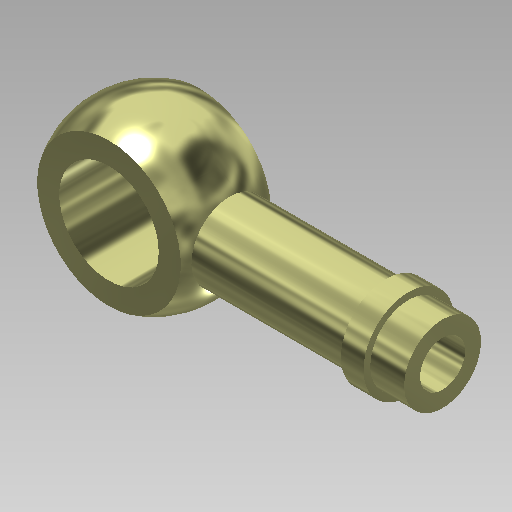
# Autodesk Inventor part: fuel_inlet
Saved by Autodesk Inventor 2018.1 (Build 221171000, 171)
## iProperties
Created: 2013-08-26
Part Number: fuel_inlet
Material: Generic
Document SubType Name: Modeling
Designer: Konstantin
Density: 1 g/cm^3
Appearance: Default
Mass: 0.152735 g
Surface Area: 3.51801 cm^2
Volume: 0.152735 cm^3
Author: Konstantin
Autodesk Inventor part; units mm, degrees
ref_plane "YZ Plane" through (0, 0, 0) normal (1, 0, 0) x (0, 1, 0)
ref_plane "XZ Plane" through (0, 0, 0) normal (0, 1, 0) x (-1, 0, 0)
ref_plane "XY Plane" through (0, 0, 0) normal (0, 0, 1) x (1, 0, 0)
sketch "Sketch2" plane through (0, 0, 0) normal (0, 0, 1) x (1, 0, 0)
  arc A0 (0, -3.75) -> (0, 3.75) centre (0, 0) ccw
  line L0 (0, -3.75) -> (0, 3.75)
  constraints: 2 end point, 2 point on circle, 1 centre point, 1 midpoint, 1 vertical, 1 other
revolve "Revolution2" add sketch "Sketch2" angle 360 about axis through (0, -3.75, 0) along (0, 1, 0)
sketch "Sketch3" plane through (0, 0, 0) normal (1, 0, 0) x (0, 1, 0)
  line L0 (4.6089, 2) -> (-4.4968, 2)
  line L1 (4.6089, -2) -> (-4.4968, -2)
  line L2 (4.6089, 5.4189) -> (-4.4968, 5.4189)
  line L3 (-4.4968, -5.0685) -> (4.6089, -5.0685)
  line L4 (4.6089, -5.0685) -> (4.6089, -2)
  line L5 (4.6089, 2) -> (4.6089, 5.4189)
  line L6 (-4.4968, 5.4189) -> (-4.4968, 2)
  line L7 (-4.4968, -2) -> (-4.4968, -5.0685)
  constraints: 16 end point, 6 horizontal, 6 parallel, 4 vertical, 2 perpendicular
extrude "Extrusion1" cut sketch "Sketch3" along normal mid plane 10
sketch "Sketch4" plane through (0, 0, 2) normal (0, 0, 1) x (1, 0, 0)
  circle A0 centre (0, 0) radius 2.2
  dimension "d8" = 4.4
  constraints: 1 centre point, 1 coincident
  measures "d8" diameter of A0
extrude "Extrusion2" cut sketch "Sketch4" against normal blind 5
sketch "Sketch5" plane through (0, 0, 0) normal (0, 0, 1) x (1, 0, 0)
  arc A0 (3.75, 0) -> (3.3425, 1.7) centre (0, 0) ccw
  line L0 (3.75, 0) -> (12.75, 0)
  line L1 (12.75, 1.7) -> (12.75, 0)
  line L2 (10.25, 2) -> (11.25, 2)
  line L3 (11.25, 2) -> (11.25, 1.7)
  line L4 (10.25, 2) -> (10.25, 1.7)
  line L5 (3.3425, 1.7) -> (10.25, 1.7)
  line L6 (11.25, 1.7) -> (12.75, 1.7)
  constraints: 14 end point, 5 horizontal, 3 parallel, 3 vertical, 2 perpendicular, 2 point on circle, 1 centre point, 1 other
revolve "Revolution3" add sketch "Sketch5" angle 360 about axis through (3.75, 0, 0) along (1, 0, 0)
sketch "Sketch6" plane through (12.75, 0, 0) normal (1, 0, 0) x (0, 0, -1)
  circle A0 centre (0, 0) radius 1
  dimension "d17" = 2
  constraints: 1 centre point, 1 coincident
  measures "d17" diameter of A0
extrude "Extrusion3" cut sketch "Sketch6" against normal blind 12
body "Solid2"
